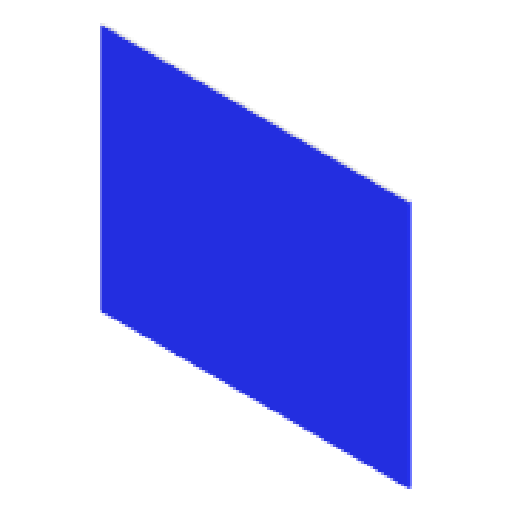
# Autodesk Inventor part: Боковая часть корпуса
Saved by Autodesk Inventor 2023.2 (Build 272271030, 271C)
## iProperties
Created: 2025-04-24
Part Number: Боковая часть корпуса
Material: Типовые
Document SubType Name: Modeling
Designer: Коноваленко
Density: 1 g/cm^3
Appearance: По умолчанию
Author: Коноваленко
Autodesk Inventor part; units mm, degrees
ref_plane "YZ Plane" through (0, 0, 0) normal (1, 0, 0) x (0, 1, 0)
ref_plane "XZ Plane" through (0, 0, 0) normal (0, 1, 0) x (-1, 0, 0)
ref_plane "XY Plane" through (0, 0, 0) normal (0, 0, 1) x (1, 0, 0)
sketch "Эскиз1" plane through (0, 0, 0) normal (0, 0, 1) x (1, 0, 0)
  line L0 (230, 185) -> (230, -185)
  line L1 (230, -185) -> (-230, -185)
  line L2 (-230, -185) -> (-230, 185)
  line L3 (-230, 185) -> (230, -185) construction
  line L4 (230, 185) -> (-230, -185) construction
  line L5 (-322, 0) -> (322, 0) construction
  line L6 (0, 259) -> (0, -259) construction
  line L7 (-230, 185) -> (230, 185)
  point P0 (0, 0)
  dimension "d2" = 370
  dimension "d4" = 460
  constraints: 12 end point, 3 perpendicular, 2 midpoint, 1 horizontal
  measures "d2" distance of L1.end L2.end
  measures "d4" distance of L0.end L1.end
extrude "Выдавливание1" add sketch "Эскиз1" along normal mid plane 4
